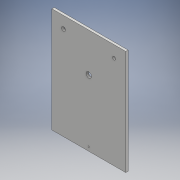
# Autodesk Inventor part: trasera
Saved by Autodesk Inventor 2018 (Build 220112000, 112)
## iProperties
Created: 2019-02-27
Part Number: trasera
Material: Genérico
Document SubType Name: Modeling
Designer: USUARIO WINDOWS
Density: 1 g/cm^3
Appearance: Valor por defecto
Author: USUARIO WINDOWS
Autodesk Inventor part; units mm, degrees
ref_plane "YZ Plane" through (0, 0, 0) normal (1, 0, 0) x (0, 1, 0)
ref_plane "XZ Plane" through (0, 0, 0) normal (0, 1, 0) x (-1, 0, 0)
ref_plane "XY Plane" through (0, 0, 0) normal (0, 0, 1) x (1, 0, 0)
sketch "Boceto1" plane through (0, 0, 0) normal (0, 1, 0) x (-1, 0, 0)
  line L0 (0, 0) -> (-105, 0)
  line L1 (-105, 0) -> (-105, -140)
  line L2 (-105, -140) -> (0, -140)
  line L3 (0, -140) -> (0, 0)
  dimension "d0" = 105
  dimension "d1" = 140
  constraints: 8 end point, 2 parallel, 1 horizontal, 1 perpendicular
  measures "d0" distance of L2.end L1.end
  measures "d1" distance of L1.end L0.end
extrude "Extrusión1" add sketch "Boceto1" along normal blind 3
sketch "Boceto2" plane through (0, 3, 0) normal (0, 1, 0) x (1, 0, 0)
  circle A0 centre (85, 15) radius 2
  circle A1 centre (20, 15) radius 2.5
  circle A2 centre (52.5, 50) radius 3.5
  line L0 (0, 0) -> (105, 0) projected
  line L1 (0, 140) -> (0, 0) projected
  line L2 (105, 0) -> (105, 140) projected
  line L3 (52.5, 50) -> (52.5, -7.4445)
  dimension "d4" = 4
  dimension "d5" = 5
  dimension "d6" = 7
  dimension "d7" = 15
  dimension "d8" = 15
  dimension "d9" = 50
  dimension "d10" = 52.5
  dimension "d11" = 105
  dimension "d14" = 85
  dimension "d15" = 85
  constraints: 3 centre point, 2 end point, 1 vertical
  measures "d4" diameter of A0
  measures "d5" diameter of A1
  measures "d6" diameter of A2
  measures "d7" distance from line of L0 A0.centre
  measures "d8" distance from line of L0 A1.centre
  measures "d9" distance from line of L0 L3.start
  measures "d10" distance from line of L1 L3.start
  measures "d11" distance between parallel lines of L2 L1
  measures "d14" distance from line of L1 A0.centre
  measures "d15" distance from line of L2 A1.centre
extrude "Extrusión2" cut sketch "Boceto2" against normal blind 3
sketch "Boceto3" plane through (0, 3, 0) normal (0, 1, 0) x (1, 0, 0)
  circle A0 centre (20, 15) radius 2.5 projected
  circle A1 centre (85, 15) radius 2 projected
  circle A2 centre (52.5, 50) radius 3.5 projected
  line L0 (0, 0) -> (105, 0) projected
  line L1 (105, 0) -> (105, 140) projected
  line L2 (105, 140) -> (0, 140) projected
  line L3 (0, 140) -> (0, 0) projected
  circle A3 centre (52.5, 130) radius 1
  dimension "d18" = 2
  dimension "d19" = 0
  dimension "d20" = 10
  constraints: 1 centre point
  measures "d18" diameter of A3
  measures "d19" horizontal distance of A2.centre A3.centre
  measures "d20" distance from line of L2 A3.centre
extrude "Extrusión3" cut sketch "Boceto3" against normal blind 3 contours A3
sketch "Boceto4" plane through (105, 0, -140) normal (0, 0, -1) x (-1, 0, 0)
  line L0 (0, 0) -> (105, 0) projected
  line L1 (105, 0) -> (105, 3) projected
  line L2 (0, 3) -> (105, 3) projected
  line L3 (0, 0) -> (0, 3) projected
extrude "Extrusión4" cut sketch "Boceto4" against normal blind 5
sketch "Boceto5" plane through (0, 3, 0) normal (0, 1, 0) x (1, 0, 0)
  line L0 (105, 135) -> (0, 135) projected
  line L1 (0, 135) -> (0, 0) projected
  line L2 (0, 0) -> (105, 0) projected
  line L3 (105, 0) -> (105, 135) projected
  circle A0 centre (52.5, 50) radius 3.5 projected
  circle A1 centre (85, 15) radius 2 projected
  circle A2 centre (20, 15) radius 2.5 projected
  circle A3 centre (52.5, 130) radius 1 projected
  line L4 (105, 135) -> (0, 135) projected
  line L5 (102.5, 0) -> (2.5, 0)
  line L6 (2.5, 0) -> (2.5, 135)
  line L7 (2.5, 135) -> (102.5, 135)
  line L8 (102.5, 135) -> (102.5, 0)
  line L9 (102.5, 0) -> (2.5, 135) construction
  line L10 (2.5, 0) -> (102.5, 135) construction
  point P0 (52.5, 67.5)
  dimension "d25" = 100
  constraints: 12 end point, 2 midpoint, 2 parallel, 1 horizontal, 1 perpendicular, 1 point on line
  measures "d25" distance of L6.end L7.end
extrude "Extrusión5" cut sketch "Boceto5" against normal blind 3 contours L3 L2 L8 L0 | L6 L2 L1 L0
sketch "Boceto6" plane through (0, 0, 0) normal (0, -1, 0) x (1, 0, 0)
  line L0 (102.5, -135) -> (102.5, 0) projected
  line L1 (2.5, 0) -> (102.5, 0) projected
  line L2 (2.5, 0) -> (2.5, -135) projected
  line L3 (2.5, -135) -> (102.5, -135) projected
  circle A0 centre (52.5, -130) radius 1 projected
  circle A1 centre (20, -15) radius 2.5 projected
  circle A2 centre (85, -15) radius 2 projected
  circle A3 centre (52.5, -50) radius 3.5 projected
  line L4 (2.5, 0) -> (102.5, 0) projected
  line L5 (100, -135) -> (5, -135)
  line L6 (5, -135) -> (5, 0)
  line L7 (5, 0) -> (100, 0)
  line L8 (100, 0) -> (100, -135)
  line L9 (100, -135) -> (5, 0) construction
  line L10 (5, -135) -> (100, 0) construction
  point P0 (0, 0)
  point P1 (52.5, -67.5)
  dimension "d28" = 95
  constraints: 12 end point, 2 midpoint, 2 parallel, 1 horizontal, 1 perpendicular, 1 point on line
  measures "d28" distance of L6.end L7.end
extrude "Extrusión6" cut sketch "Boceto6" against normal blind 3 contours L3 L8 L1 L0 | L3 L2 L1 L6
equation "\"d10\" = 0.5 * d11"
